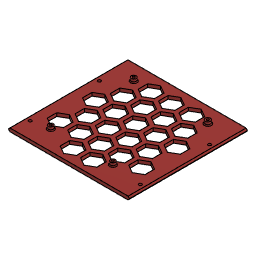
MCU Tray - BTT SKR 3 EZ (Autodesk Fusion 360 design; units mm, degrees)
Autodesk Fusion 360 part; units mm, degrees
note: some values were not read from the file. Chosen so that the rebuilt part matches the saved one: a direction.
imported_body "Derived Base Feature2" makes body 1
imported_body "Derived Base Feature1" makes body 2
sketch "Base Profile" plane through (0, 0, 0) normal (0, 1, 0) x (1, 0, 0)
  line L0 (72.5, 2) -> (-72.5, 2)
  line L1 (-72.5, 2) -> (-72.5, -2) construction
  line L2 (-72.5, -2) -> (72.5, -2)
  line L3 (72.5, -2) -> (72.5, 2) construction
  line L4 (72.5, 2) -> (-72.5, -2) construction
  line L5 (-72.5, 2) -> (72.5, -2) construction
  line L6 (-72.5, 0) -> (-74.3, 0) construction
  line L7 (-72.5, -2) -> (-74.3, -0.2)
  line L8 (-74.3, 0.2) -> (-72.5, 2)
  line L9 (-74.3, -0.2) -> (-74.3, 0)
  line L10 (-74.3, 0) -> (-74.3, 0.2)
  line L11 (0, 0) -> (0, -2) construction
  line L12 (72.5, -2) -> (74.3, -0.2)
  line L13 (74.3, -0.2) -> (74.3, 0)
  line L14 (74.3, 0) -> (74.3, 0.2)
  line L15 (74.3, 0.2) -> (72.5, 2)
  dimension "d1" = 145
  dimension "d2" = 4
  dimension "d3" = 0.2
  constraint horizontal L0
  constraint perpendicular L0 L1
  constraint parallel L0 L2
  constraint parallel L1 L3
  constraint coincident L4 L11.start
  constraint coincident L5 L11.start
  constraint coincident L11.start origin
  constraint midpoint L1 L6.start
  constraint perpendicular L1 L6
  constraint coincident L5 L0.end
  constraint coincident L0 L1.start
  constraint perpendicular L6 L9
  constraint perpendicular L6 L10
  constraint midpoint L2 L11.end
  constraint symmetric L1.end L11 L2.end
  constraint symmetric L0.end L11 L0.start
  constraint symmetric L7.end L11 L12.end
  constraint symmetric L6.end L11 L13.end
  constraint symmetric L8.start L11 L14.end
  measures "d1" distance of L1.end L2.end
  measures "d2" distance of L0.end L1.end
  measures "d3" distance of L7.end L6.end
extrude "Extrude1" add sketch "Base Profile" along normal blind 190 and the other way blind 15 separate body makes body 3
sketch "M3 Mount Holes" plane through (0, 0, 2) normal (0, 0, 1) x (-1, 0, 0)
  line L0 (72.5, 15) -> (-72.5, 15)
  line L1 (-72.5, 15) -> (-72.5, -190)
  line L2 (-72.5, -190) -> (72.5, -190)
  line L3 (72.5, -190) -> (72.5, 15)
  line L4 (0, 0) -> (0, -13.0831) construction
  circle A0 centre (-67.6414, -5) radius 1.8
  line L5 (72.6414, -59.8458) -> (72.6414, 0.0002) construction
  circle A1 centre (67.6414, -5) radius 1.8
  line L6 (72.5, -190) -> (72.5, 15)
  line L7 (72.6414, 0.0002) -> (78.5, 0.0002)
  line L8 (67.6414, -5) -> (72.6414, -5) construction
  line L9 (72.6414, -5) -> (72.6414, 0.0002) construction
  line L10 (67.6414, -5) -> (67.6414, -90) construction
  circle A2 centre (67.6414, -90) radius 1.8
  circle A3 centre (-67.6414, -90) radius 1.8
  dimension "d16" = 3.6
  dimension "d17" = 85
  dimension "d18" = 3.6
  dimension "d42" = 5
  dimension "d43" = 20
  constraint coincident L4.start origin
  constraint vertical L4
  constraint symmetric L4 A0 A1
  constraint horizontal L8
  constraint vertical L9
  constraint coincident L5.end L7.start
  constraint coincident A1.centre L8.start
  constraint perpendicular L8 L10
  constraint coincident L10.end A2.centre
  constraint symmetric L4 A2 A3
  measures "d16" diameter of A1
  measures "d17" distance of A1.centre L10.end
  measures "d18" diameter of A2
  measures "d42" distance of A1.centre L8.end
  measures "d43" distance of L0 A1.centre
sketch "M4 Mount Holes" plane through (0, 0, 2) normal (0, 0, 1) x (-1, 0, 0)
  line L0 (-72.5, 15) -> (-72.5, -190)
  line L1 (-72.5, -190) -> (72.5, -190)
  line L2 (72.5, -190) -> (72.5, 15)
  line L3 (72.5, 15) -> (-72.5, 15)
  circle A0 centre (-67.6414, -5) radius 1.8 construction
  circle A1 centre (-67.6414, -5) radius 2.3
  line L4 (-67.6414, -5) -> (-67.6414, -90) construction
  circle A2 centre (-67.6414, -90) radius 2.3
  line L5 (0, 0) -> (0, -24.5368) construction
  circle A3 centre (67.6414, -90) radius 2.3
  circle A4 centre (67.6414, -5) radius 2.3
  dimension "d37" = 4.6
  dimension "d38" = 85
  dimension "d39" = 4.6
  constraint concentric A0 A1
  constraint coincident A0.centre A1.centre
  constraint parallel L0 L4
  constraint coincident L4.end A2.centre
  constraint coincident L5.start origin
  constraint vertical L5
  constraint symmetric A1 L5 A4
  constraint symmetric A2 L5 A3
  measures "d37" diameter of A1
  measures "d38" distance of A0.centre L4.end
  measures "d39" diameter of A2
extrude "Extrude2" cut sketch "M3 Mount Holes" against normal up to surface (4 mm away) contours A0 | A1 | A2 | A3 bodies 3
extrude "Extrude5" [suppressed]
extrude "Extrude3" cut 1 faces at (24.1667, 190, 0.6667) along direction (0, -1, 0) blind 40.154 on bodies 3 bodies 3
delete_body "RemoveBody1" bodies 2
delete_body "RemoveBody2" bodies 1
sketch "Vent Holes" plane through (0, 0, 2) normal (0, 0, 1) x (-1, 0, 0)
  line L0 (-72.5, -149.846) -> (72.5, -149.846)
  line L1 (72.5, -149.846) -> (72.5, 15)
  line L2 (72.5, 15) -> (-72.5, 15)
  line L3 (-72.5, 15) -> (-72.5, -149.846)
  line L4 (0, 15) -> (0, -149.846) construction
  line L5 (10, -61.6495) -> (0, -55.876)
  line L6 (0, -55.876) -> (-10, -61.6495)
  line L7 (-10, -61.6495) -> (-10, -73.1965)
  line L8 (-10, -73.1965) -> (0, -78.97)
  line L9 (0, -78.97) -> (10, -73.1965)
  line L10 (10, -73.1965) -> (10, -61.6495)
  line L11 (0, -67.423) -> (5, -76.0833) construction
  line L12 (0, -67.423) -> (-5, -76.0833) construction
  line L13 (10, -73.1965) -> (10, -61.6495)
  line L14 (10, -61.6495) -> (0, -55.876)
  line L15 (0, -55.876) -> (-10, -61.6495)
  line L16 (-10, -61.6495) -> (-10, -73.1965)
  line L17 (-10, -73.1965) -> (0, -78.97)
  line L18 (0, -78.97) -> (10, -73.1965)
  line L19 (-15, -18.3482) -> (-25, -12.5747)
  line L20 (-25, -12.5747) -> (-35, -18.3482)
  line L21 (-35, -18.3482) -> (-35, -29.8952)
  line L22 (-35, -29.8952) -> (-25, -35.6687)
  line L23 (-25, -35.6687) -> (-15, -29.8952)
  line L24 (-15, -29.8952) -> (-15, -18.3482)
  line L25 (-27.5, 3.3024) -> (-37.5, 9.0759)
  line L26 (-37.5, 9.0759) -> (-47.5, 3.3024)
  line L27 (-47.5, 3.3024) -> (-47.5, -8.2446)
  line L28 (-47.5, -8.2446) -> (-37.5, -14.0181)
  line L29 (-37.5, -14.0181) -> (-27.5, -8.2446)
  line L30 (-27.5, -8.2446) -> (-27.5, 3.3024)
  line L31 (-2.5, -39.9989) -> (-12.5, -34.2254)
  line L32 (-12.5, -34.2254) -> (-22.5, -39.9989)
  line L33 (-22.5, -39.9989) -> (-22.5, -51.5459)
  line L34 (-22.5, -51.5459) -> (-12.5, -57.3194)
  line L35 (-12.5, -57.3194) -> (-2.5, -51.5459)
  line L36 (-2.5, -51.5459) -> (-2.5, -39.9989)
  line L37 (22.5, -83.3001) -> (12.5, -77.5266)
  line L38 (12.5, -77.5266) -> (2.5, -83.3001)
  line L39 (2.5, -83.3001) -> (2.5, -94.8471)
  line L40 (2.5, -94.8471) -> (12.5, -100.6206)
  line L41 (12.5, -100.6206) -> (22.5, -94.8471)
  line L42 (22.5, -94.8471) -> (22.5, -83.3001)
  line L43 (35, -104.9508) -> (25, -99.1773)
  line L44 (25, -99.1773) -> (15, -104.9508)
  line L45 (15, -104.9508) -> (15, -116.4978)
  line L46 (15, -116.4978) -> (25, -122.2713)
  line L47 (25, -122.2713) -> (35, -116.4978)
  line L48 (35, -116.4978) -> (35, -104.9508)
  line L49 (47.5, -126.6014) -> (37.5, -120.8279)
  line L50 (37.5, -120.8279) -> (27.5, -126.6014)
  line L51 (27.5, -126.6014) -> (27.5, -138.1484)
  line L52 (27.5, -138.1484) -> (37.5, -143.9219)
  line L53 (37.5, -143.9219) -> (47.5, -138.1484)
  line L54 (47.5, -138.1484) -> (47.5, -126.6014)
  line L55 (12.5, -57.3194) -> (22.5, -51.5459)
  line L56 (22.5, -51.5459) -> (22.5, -39.9989)
  line L57 (22.5, -39.9989) -> (12.5, -34.2254)
  line L58 (12.5, -34.2254) -> (2.5, -39.9989)
  line L59 (2.5, -51.5459) -> (12.5, -57.3194)
  line L60 (2.5, -39.9989) -> (2.5, -51.5459)
  line L61 (-15, -61.6495) -> (-25, -55.876)
  line L62 (-25, -55.876) -> (-35, -61.6495)
  line L63 (-35, -61.6495) -> (-35, -73.1965)
  line L64 (-35, -73.1965) -> (-25, -78.97)
  line L65 (-15, -73.1965) -> (-15, -61.6495)
  line L66 (-25, -78.97) -> (-15, -73.1965)
  line L67 (-2.5, 3.3024) -> (-12.5, 9.0759)
  line L68 (-12.5, 9.0759) -> (-22.5, 3.3024)
  line L69 (-22.5, 3.3024) -> (-22.5, -8.2446)
  line L70 (-22.5, -8.2446) -> (-12.5, -14.0181)
  line L71 (-12.5, -14.0181) -> (-2.5, -8.2446)
  line L72 (-2.5, -8.2446) -> (-2.5, 3.3024)
  line L73 (-40, -18.3482) -> (-50, -12.5747)
  line L74 (-50, -12.5747) -> (-60, -18.3482)
  line L75 (-60, -18.3482) -> (-60, -29.8952)
  line L76 (-60, -29.8952) -> (-50, -35.6687)
  line L77 (-40, -29.8952) -> (-40, -18.3482)
  line L78 (-50, -35.6687) -> (-40, -29.8952)
  line L79 (10, -18.3482) -> (0, -12.5747)
  line L80 (0, -12.5747) -> (-10, -18.3482)
  line L81 (-10, -18.3482) -> (-10, -29.8952)
  line L82 (-10, -29.8952) -> (0, -35.6687)
  line L83 (0, -35.6687) -> (10, -29.8952)
  line L84 (10, -29.8952) -> (10, -18.3482)
  line L85 (-27.5, -39.9989) -> (-37.5, -34.2254)
  line L86 (-37.5, -34.2254) -> (-47.5, -39.9989)
  line L87 (-47.5, -39.9989) -> (-47.5, -51.5459)
  line L88 (-47.5, -51.5459) -> (-37.5, -57.3194)
  line L89 (-27.5, -51.5459) -> (-27.5, -39.9989)
  line L90 (-37.5, -57.3194) -> (-27.5, -51.5459)
  line L91 (35, -61.6495) -> (25, -55.876)
  line L92 (25, -55.876) -> (15, -61.6495)
  line L93 (15, -61.6495) -> (15, -73.1965)
  line L94 (15, -73.1965) -> (25, -78.97)
  line L95 (25, -78.97) -> (35, -73.1965)
  line L96 (35, -73.1965) -> (35, -61.6495)
  line L97 (-2.5, -83.3001) -> (-12.5, -77.5266)
  line L98 (-12.5, -77.5266) -> (-22.5, -83.3001)
  line L99 (-22.5, -83.3001) -> (-22.5, -94.8471)
  line L100 (-22.5, -94.8471) -> (-12.5, -100.6206)
  line L101 (-2.5, -94.8471) -> (-2.5, -83.3001)
  line L102 (-12.5, -100.6206) -> (-2.5, -94.8471)
  line L103 (47.5, -83.3001) -> (37.5, -77.5266)
  line L104 (37.5, -77.5266) -> (27.5, -83.3001)
  line L105 (27.5, -83.3001) -> (27.5, -94.8471)
  line L106 (27.5, -94.8471) -> (37.5, -100.6206)
  line L107 (37.5, -100.6206) -> (47.5, -94.8471)
  line L108 (47.5, -94.8471) -> (47.5, -83.3001)
  line L109 (10, -104.9508) -> (0, -99.1773)
  line L110 (0, -99.1773) -> (-10, -104.9508)
  line L111 (-10, -104.9508) -> (-10, -116.4978)
  line L112 (-10, -116.4978) -> (0, -122.2713)
  line L113 (10, -116.4978) -> (10, -104.9508)
  line L114 (0, -122.2713) -> (10, -116.4978)
  line L115 (60, -104.9508) -> (50, -99.1773)
  line L116 (50, -99.1773) -> (40, -104.9508)
  line L117 (40, -104.9508) -> (40, -116.4978)
  line L118 (40, -116.4978) -> (50, -122.2713)
  line L119 (50, -122.2713) -> (60, -116.4978)
  line L120 (60, -116.4978) -> (60, -104.9508)
  line L121 (22.5, -126.6014) -> (12.5, -120.8279)
  line L122 (12.5, -120.8279) -> (2.5, -126.6014)
  line L123 (2.5, -126.6014) -> (2.5, -138.1484)
  line L124 (2.5, -138.1484) -> (12.5, -143.9219)
  line L125 (22.5, -138.1484) -> (22.5, -126.6014)
  line L126 (12.5, -143.9219) -> (22.5, -138.1484)
  line L127 (-47.5, -45.7724) -> (-60, -45.7724) construction
  line L128 (-40, -61.6495) -> (-40, -73.1965)
  line L129 (-40, -73.1965) -> (-50, -78.97)
  line L130 (-50, -78.97) -> (-60, -73.1965)
  line L131 (-60, -73.1965) -> (-60, -61.6495)
  line L132 (-60, -61.6495) -> (-50, -55.876)
  line L133 (-50, -55.876) -> (-40, -61.6495)
  line L134 (47.5, -89.0736) -> (60, -89.0736) construction
  line L135 (40, -73.1965) -> (40, -61.6495)
  line L136 (40, -61.6495) -> (50, -55.876)
  line L137 (50, -55.876) -> (60, -61.6495)
  line L138 (60, -61.6495) -> (60, -73.1965)
  line L139 (60, -73.1965) -> (50, -78.97)
  line L140 (50, -78.97) -> (40, -73.1965)
  line L141 (-47.5, -94.8471) -> (-47.5, -83.3001)
  line L142 (-47.5, -83.3001) -> (-37.5, -77.5266)
  line L143 (-37.5, -77.5266) -> (-27.5, -83.3001)
  line L144 (-27.5, -83.3001) -> (-27.5, -94.8471)
  line L145 (-27.5, -94.8471) -> (-37.5, -100.6206)
  line L146 (-37.5, -100.6206) -> (-47.5, -94.8471)
  line L147 (-60, -116.4978) -> (-60, -104.9508)
  line L148 (-60, -104.9508) -> (-50, -99.1773)
  line L149 (-50, -99.1773) -> (-40, -104.9508)
  line L150 (-40, -104.9508) -> (-40, -116.4978)
  line L151 (-50, -122.2713) -> (-60, -116.4978)
  line L152 (-40, -116.4978) -> (-50, -122.2713)
  line L153 (-27.5, -126.6014) -> (-27.5, -138.1484)
  line L154 (-27.5, -138.1484) -> (-37.5, -143.9219)
  line L155 (-37.5, -143.9219) -> (-47.5, -138.1484)
  line L156 (-47.5, -138.1484) -> (-47.5, -126.6014)
  line L157 (-37.5, -120.8279) -> (-27.5, -126.6014)
  line L158 (-47.5, -126.6014) -> (-37.5, -120.8279)
  line L159 (-35, -104.9508) -> (-25, -99.1773)
  line L160 (-25, -99.1773) -> (-15, -104.9508)
  line L161 (-15, -104.9508) -> (-15, -116.4978)
  line L162 (-15, -116.4978) -> (-25, -122.2713)
  line L163 (-35, -116.4978) -> (-35, -104.9508)
  line L164 (-25, -122.2713) -> (-35, -116.4978)
  line L165 (27.5, -39.9989) -> (37.5, -34.2254)
  line L166 (37.5, -34.2254) -> (47.5, -39.9989)
  line L167 (47.5, -39.9989) -> (47.5, -51.5459)
  line L168 (47.5, -51.5459) -> (37.5, -57.3194)
  line L169 (27.5, -51.5459) -> (27.5, -39.9989)
  line L170 (37.5, -57.3194) -> (27.5, -51.5459)
  line L171 (15, -18.3482) -> (25, -12.5747)
  line L172 (25, -12.5747) -> (35, -18.3482)
  line L173 (35, -18.3482) -> (35, -29.8952)
  line L174 (35, -29.8952) -> (25, -35.6687)
  line L175 (15, -29.8952) -> (15, -18.3482)
  line L176 (25, -35.6687) -> (15, -29.8952)
  line L177 (27.5, 3.3024) -> (37.5, 9.0759)
  line L178 (37.5, 9.0759) -> (47.5, 3.3024)
  line L179 (47.5, 3.3024) -> (47.5, -8.2446)
  line L180 (47.5, -8.2446) -> (37.5, -14.0181)
  line L181 (27.5, -8.2446) -> (27.5, 3.3024)
  line L182 (37.5, -14.0181) -> (27.5, -8.2446)
  line L183 (40, -18.3482) -> (50, -12.5747)
  line L184 (50, -12.5747) -> (60, -18.3482)
  line L185 (60, -18.3482) -> (60, -29.8952)
  line L186 (60, -29.8952) -> (50, -35.6687)
  line L187 (40, -29.8952) -> (40, -18.3482)
  line L188 (50, -35.6687) -> (40, -29.8952)
  line L189 (22.5, 3.3024) -> (22.5, -8.2446)
  line L190 (22.5, -8.2446) -> (12.5, -14.0181)
  line L191 (12.5, -14.0181) -> (2.5, -8.2446)
  line L192 (2.5, -8.2446) -> (2.5, 3.3024)
  line L193 (12.5, 9.0759) -> (22.5, 3.3024)
  line L194 (2.5, 3.3024) -> (12.5, 9.0759)
  line L195 (-2.5, -126.6014) -> (-2.5, -138.1484)
  line L196 (-2.5, -138.1484) -> (-12.5, -143.9219)
  line L197 (-12.5, -143.9219) -> (-22.5, -138.1484)
  line L198 (-22.5, -138.1484) -> (-22.5, -126.6014)
  line L199 (-12.5, -120.8279) -> (-2.5, -126.6014)
  line L200 (-22.5, -126.6014) -> (-12.5, -120.8279)
  circle A0 centre (-67.6414, -90) radius 1.8
  circle A1 centre (-67.6414, -5) radius 1.8
  circle A2 centre (67.6414, -90) radius 1.8
  circle A3 centre (67.6414, -5) radius 1.8
  point P0 (0, -67.423)
  dimension "d19" = 10
  dimension "d22" = 25
  dimension "d23" = 50
  dimension "d29" = 360
  dimension "d32" = 25
  dimension "d33" = 0
  constraint midpoint L2 L4.start
  constraint midpoint L0 L4.end
  constraint midpoint L4 P0
  constraint coincident P0 L11.start
  constraint midpoint L9 L11.end
  constraint midpoint L8 L12.end
  constraint midpoint L87 L127.start
  constraint perpendicular L87 L127
  constraint symmetric L73.start L127 L128.end
  constraint symmetric L73.end L127 L129.end
  constraint symmetric L74.end L127 L130.end
  constraint symmetric L75.end L127 L131.end
  constraint symmetric L76.end L127 L132.end
  constraint symmetric L77.start L127 L128.start
  constraint midpoint L108 L134.start
  constraint perpendicular L108 L134
  constraint symmetric L115.start L134 L138.end
  constraint symmetric L115.end L134 L139.end
  constraint symmetric L116.end L134 L135.start
  constraint symmetric L117.end L134 L135.end
  constraint symmetric L118.end L134 L136.end
  constraint symmetric L119.end L134 L137.end
  constraint symmetric L4 L19.start L171.start
  constraint symmetric L4 L19.end L171.end
  constraint symmetric L4 L20.end L172.end
  constraint symmetric L4 L21.end L173.end
  constraint symmetric L4 L22.end L174.end
  constraint symmetric L4 L23.end L175.start
  constraint symmetric L4 L25.start L177.start
  constraint symmetric L4 L25.end L177.end
  constraint symmetric L4 L26.end L178.end
  constraint symmetric L4 L27.end L179.end
  constraint symmetric L4 L28.end L180.end
  constraint symmetric L4 L29.end L181.start
  constraint symmetric L4 L43.start L159.start
  constraint symmetric L4 L43.end L159.end
  constraint symmetric L4 L44.end L160.end
  constraint symmetric L4 L45.end L161.end
  constraint symmetric L4 L46.end L162.end
  constraint symmetric L4 L47.end L163.start
  constraint symmetric L4 L49.start L156.end
  constraint symmetric L4 L49.end L157.start
  constraint symmetric L4 L50.end L153.start
  constraint symmetric L4 L51.end L153.end
  constraint symmetric L4 L52.end L154.end
  constraint symmetric L4 L53.end L155.end
  constraint symmetric L4 L67.start L192.end
  constraint symmetric L4 L67.end L193.start
  constraint symmetric L4 L68.end L189.start
  constraint symmetric L4 L69.end L189.end
  constraint symmetric L4 L70.end L190.end
  constraint symmetric L4 L71.end L191.end
  constraint symmetric L4 L73.start L183.start
  constraint symmetric L4 L73.end L183.end
  constraint symmetric L4 L74.end L184.end
  constraint symmetric L4 L75.end L185.end
  constraint symmetric L4 L76.end L186.end
  constraint symmetric L4 L77.start L187.start
  constraint symmetric L4 L85.start L165.start
  constraint symmetric L4 L85.end L165.end
  constraint symmetric L4 L86.end L166.end
  constraint symmetric L4 L87.end L167.end
  constraint symmetric L4 L88.end L168.end
  constraint symmetric L4 L89.start L169.start
  constraint symmetric L4 L103.start L141.end
  constraint symmetric L4 L103.end L142.end
  constraint symmetric L4 L104.end L143.end
  constraint symmetric L4 L105.end L144.end
  constraint symmetric L4 L106.end L145.end
  constraint symmetric L4 L107.end L141.start
  constraint symmetric L4 L115.start L147.end
  constraint symmetric L4 L115.end L148.end
  constraint symmetric L4 L116.end L149.end
  constraint symmetric L4 L117.end L150.end
  constraint symmetric L4 L118.end L151.start
  constraint symmetric L4 L119.end L147.start
  constraint symmetric L4 L121.start L198.end
  constraint symmetric L4 L121.end L199.start
  constraint symmetric L4 L122.end L195.start
  constraint symmetric L4 L123.end L195.end
  constraint symmetric L4 L124.end L196.end
  constraint symmetric L4 L125.start L197.end
  measures "d19" distance of P0 L10
sketch "Sketch5" plane through (0, 0, 2) normal (0, 0, 1) x (-1, 0, 0)
  line L0 (-72.5, -149.846) -> (72.5, -149.846)
  line L1 (72.5, -149.846) -> (72.5, 15)
  line L2 (72.5, 15) -> (-72.5, 15)
  line L3 (-72.5, 15) -> (-72.5, -149.846)
  circle A0 centre (-67.6414, -90) radius 1.8
  circle A1 centre (-67.6414, -5) radius 1.8
  circle A2 centre (67.6414, -90) radius 1.8
  circle A3 centre (67.6414, -5) radius 1.8
  line L4 (50.5231, -113.8025) -> (50.5231, -6.289) construction
  circle A4 centre (46.548, -111.0301) radius 1.7272 construction
  line L5 (49.5106, -5.3241) -> (-46.2115, -5.3241) construction
  arc A5 (49.4036, -114.9941) -> (50.5231, -113.8025) centre (49.3281, -113.8015) ccw construction
  circle A6 centre (-44.2468, -111.1738) radius 1.65 construction
  line L6 (-46.1044, -114.9941) -> (49.4036, -114.9941) construction
  circle A7 centre (-29.7568, -9.1801) radius 1.7272 construction
  line L7 (-47.4769, -6.606) -> (-47.4769, -113.7015) construction
  arc A8 (-46.2115, -5.3241) -> (-47.4769, -6.606) centre (-46.1949, -6.6061) ccw construction
  arc A9 (50.5231, -6.289) -> (49.5106, -5.3241) centre (49.5569, -6.2892) ccw construction
  circle A10 centre (46.548, -9.1801) radius 1.7272 construction
  arc A11 (-47.4769, -113.7015) -> (-46.1044, -114.9941) centre (-46.1829, -113.7025) ccw construction
  line L8 (1.6496, -114.9941) -> (1.6496, -5.3241) construction
  line L9 (46.548, -9.1801) -> (-29.7568, -9.1801) construction
  line L10 (46.548, -111.0301) -> (46.548, -9.1801) construction
  line L11 (-29.7568, -9.1801) -> (-47.4769, -9.1801) construction
  line L12 (-44.2468, -111.1738) -> (-44.2468, -9.1801) construction
  line L13 (-44.2468, -111.1738) -> (-47.4769, -111.1738) construction
  line L14 (46.548, -111.0301) -> (50.5231, -111.0301) construction
  circle A12 centre (-29.7568, -9.1801) radius 1.4
  circle A13 centre (-29.7568, -9.1801) radius 3
  circle A14 centre (46.548, -9.1801) radius 1.4
  circle A15 centre (46.548, -9.1801) radius 3
  circle A16 centre (-44.2468, -111.1738) radius 1.4
  circle A17 centre (-44.2468, -111.1738) radius 3.25
  circle A18 centre (46.548, -111.0301) radius 1.4
  circle A19 centre (46.548, -111.0301) radius 3
  point P0 (50.5231, -114.9965)
  dimension "d44" = 98
  dimension "d45" = 109.67
  dimension "d46" = 101.85
  dimension "d47" = 14.49
  dimension "d48" = 3.2301
  dimension "d49" = 3.9751
  dimension "d50" = 2.8
  dimension "d51" = 1.6
  dimension "d52" = 2.8
  dimension "d53" = 1.6
  dimension "d54" = 2.8
  dimension "d55" = 1.6
  dimension "d56" = 2.8
  dimension "d57" = 1.6
  constraint midpoint L6 L8.start
  constraint midpoint L5 L8.end
  constraint coincident A10.centre L9.start
  constraint coincident A7.centre L9.end
  constraint coincident A4.centre L10.start
  constraint perpendicular L6 L10
  constraint coincident L7 L11.end
  constraint perpendicular L7 L11
  constraint coincident A6.centre L12.start
  constraint coincident L11 L12.end
  constraint perpendicular L11 L12
  constraint vertical L12
  constraint vertical L10
  constraint horizontal L9
  constraint vertical L8
  constraint coincident L7 L13.end
  constraint perpendicular L7 L13
  constraint coincident L4 L14.end
  constraint perpendicular L4 L14
  measures "d44" distance of L4 L7
  measures "d45" distance of L5 L6
  measures "d46" distance of A10.centre A4.centre
  measures "d47" distance of A7.centre L12
  measures "d48" distance of A6.centre L13.end
  measures "d49" distance of A4.centre L14.end
  measures "d50" diameter of A12
  measures "d52" diameter of A14
  measures "d54" diameter of A16
  measures "d56" diameter of A18
extrude "Extrude6" add sketch "Sketch5" along normal blind 4 contours A13 | A15 | A17 | A19 bodies 3
extrude "Extrude7" cut sketch "Sketch5" against normal blind 4 contours A12 | A14 | A16 | A18 bodies 3
fillet "Fillet1" radius 1 4 edges at (47.2768, 109.9986, 2) (-43.751, 109.9453, 2) (-43.751, 8.0953, 2) (32.5538, 8.0953, 2) on bodies 3
extrude "Extrude4" cut sketch "Vent Holes" against normal blind 8 contours L5 L6 L7 L8 L9 L10 L13 L14 L15 L16 L17 L18 | L19 L20 L21 L22 L23 L24 | L31 L32 L33 L34 L35 L36 | L37 L38 L39 L40 L41 L42 | L43 L44 L45 L46 L47 L48 | L55 L56 L57 L58 L59 L60 | L61 L62 L63 L64 L65 L66 | L67 L68 L69 L70 L71 L72 | L73 L74 L75 L76 L77 L78 | L79 L80 L81 L82 L83 L84 | L85 L86 L87 L88 L89 L90 | L91 L92 L93 L94 L95 L96 | L97 L98 L99 L100 L101 L102 | L103 L104 L105 L106 L107 L108 | L109 L110 L111 L112 L113 L114 | L128 L129 L130 L131 L132 L133 | L135 L136 L137 L138 L139 L140 | L141 L142 L143 L144 L145 L146 | L159 L160 L161 L162 L163 L164 | L165 L166 L167 L168 L169 L170 | L171 L172 L173 L174 L175 L176 | L183 L184 L185 L186 L187 L188 | L189 L190 L191 L192 L193 L194 bodies 3
extrude "Extrude8" cut 1 faces at (24.1667, 149.846, 0.6667) along direction (0, -1, 0) blind 20 on bodies 3 bodies 3
equation "d18 = d16"
named bodies: "Body1 (Context1)", "Body1 (Context2)"
